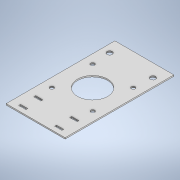
# Autodesk Inventor part: Platte1
Saved by Autodesk Inventor 2022 (Build 260153000, 153)
## iProperties
Created: 2022-04-02
Part Number: Platte1
Material: Generic
Document SubType Name: Modeling
Designer: benni
Density: 1 g/cm^3
Appearance: Default
Author: benni
Autodesk Inventor part; units mm, degrees
ref_plane "YZ Plane" through (0, 0, 0) normal (1, 0, 0) x (0, 1, 0)
ref_plane "XZ Plane" through (0, 0, 0) normal (0, 1, 0) x (-1, 0, 0)
ref_plane "XY Plane" through (0, 0, 0) normal (0, 0, 1) x (1, 0, 0)
sketch "Sketch1" plane through (0, 0, 0) normal (0, 1, 0) x (-1, 0, 0)
  line L0 (0, 0) -> (45, 0)
  line L1 (45, 0) -> (45, -83)
  line L2 (45, -83) -> (0, -83)
  line L3 (0, -83) -> (0, 0)
  circle A0 centre (39, -73) radius 2
  line L4 (22.5, 0) -> (22.5, -83)
  circle A1 centre (22.5, -43.5) radius 11.5
  circle A2 centre (38.1, -28) radius 1.5
  circle A3 centre (38, -59) radius 1.5
  circle A4 centre (6, -73) radius 2
  circle A5 centre (6.9, -28) radius 1.5
  circle A6 centre (7, -59) radius 1.5
  line L5 (45, -10) -> (0, -10)
  line L6 (6, -3.5) -> (11.525, -3.5)
  line L7 (11.525, -3.5) -> (11.525, -5)
  line L8 (11.525, -5) -> (6, -5)
  line L9 (6, -5) -> (6, -3.5)
  line L10 (6, -16.5) -> (11.525, -16.5)
  line L11 (11.525, -16.5) -> (11.525, -15)
  line L12 (11.525, -15) -> (6, -15)
  line L13 (6, -15) -> (6, -16.5)
  line L14 (39, -3.5) -> (33.475, -3.5)
  line L15 (33.475, -3.5) -> (33.475, -5)
  line L16 (33.475, -5) -> (39, -5)
  line L17 (39, -5) -> (39, -3.5)
  line L18 (39, -16.5) -> (33.475, -16.5)
  line L19 (33.475, -15) -> (39, -15)
  line L20 (39, -15) -> (39, -16.5)
  line L21 (33.475, -16.5) -> (33.475, -15)
  dimension "d0" = 45
  dimension "d1" = 83
  dimension "d2" = 10
  dimension "d3" = 6
  dimension "d9" = 4
  dimension "d13" = 45
  dimension "d14" = 24
  dimension "d15" = 31
  dimension "d16" = 31
  dimension "d17" = 15.5
  dimension "d18" = 23
  dimension "d19" = 3
  dimension "d20" = 3
  dimension "d22" = 20
  dimension "d23" = 6
  dimension "d24" = 10
  dimension "d25" = 1.5
  constraints: 44 end point, 15 symmetric about line, 7 centre point, 4 coincident, 4 parallel, 4 perpendicular, 3 point on line, 2 horizontal, 2 midpoint, 3 other
  measures "d0" distance of L1.end L2.end
  measures "d1" distance of L0.end L1.end
  measures "d2" distance from line of L2 point (39, -73)
  measures "d3" distance from line of L1 point (39, -73)
  measures "d9" diameter of A0
  measures "d13" diameter of L3 L4
  measures "d14" distance from line of L2 point (38, -59)
  measures "d15" diameter of point (38, -59) L4
  measures "d16" vertical distance of point (38, -59) point (38.1, -28)
  measures "d17" horizontal distance of point (38, -59) point (22.5, -43.5)
  measures "d18" diameter of A1
  measures "d19" diameter of A2
  measures "d20" diameter of A3
  measures "d22" diameter of L0 L5
  measures "d23" distance between parallel lines of L3 L9
  measures "d24" diameter of L8 L5
  measures "d25" distance of L6.end L7.end
extrude "Extrusion2" add sketch "Sketch1" along normal blind 1 contours L0 L4 L5 L3 | L0 L1 L5 L4 | L5 L4 A1 L2 L3 | L5 L1 L2 L4 A1
equation "\"d13\" = d0"
equation "\"d16\" = d15"
equation "\"d17\" = 0.5 * d15"
body "Solid2"
